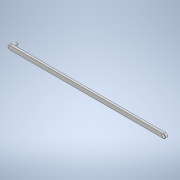
# Autodesk Inventor part: eslabon_1
Saved by Autodesk Inventor 2021 (Build 250183000, 183)
## iProperties
Created: 2021-07-12
Part Number: eslabon_1
Material: Genérico
Document SubType Name: Modeling
Designer: Leonardo Fabio Mercado Benítez
Density: 1 g/cm^3
Appearance: Valor por defecto
Author: Leonardo Fabio Mercado Benítez
Autodesk Inventor part; units mm, degrees
ref_plane "YZ Plane" through (0, 0, 0) normal (1, 0, 0) x (0, 1, 0)
ref_plane "XZ Plane" through (0, 0, 0) normal (0, 1, 0) x (-1, 0, 0)
ref_plane "XY Plane" through (0, 0, 0) normal (0, 0, 1) x (1, 0, 0)
sketch "Boceto1" plane through (0, 0, 0) normal (0, 0, 1) x (1, 0, 0)
  arc A0 (0, 3.175) -> (0, -3.175) centre (0, 0) ccw
  arc A1 (240, -3.175) -> (240, 3.175) centre (240, 0) ccw
  line L0 (0, 3.175) -> (240, 3.175)
  line L1 (240, -3.175) -> (0, -3.175)
  dimension "d0" = 6.35
  dimension "d3" = 6.35
  constraints: 4 end point, 4 point on circle, 3 tangent, 2 centre point, 1 coincident
  measures "d0" diameter of A0
  measures "d3" diameter of A1
extrude "Extrusión1" add sketch "Boceto1" along normal blind 3.175
sketch "Boceto2" plane through (0, 0, 0) normal (0, 0, -1) x (-1, 0, 0)
  circle A0 centre (0, 0) radius 2.175
  constraints: 1 centre point, 1 coincident
extrude "Extrusión2" add sketch "Boceto2" along normal blind 7
sketch "Boceto3" plane through (0, 0, 3.175) normal (0, 0, 1) x (1, 0, 0)
  arc A0 (240, -3.175) -> (240, 3.175) centre (240, 0) ccw projected
  circle A1 centre (240, 0) radius 3.175
  circle A2 centre (240, 0) radius 2.675
  point P0 (0, 0)
  dimension "d10" = 6.35
  dimension "d11" = 0.5
  constraints: 2 centre point, 1 coincident
  measures "d10" diameter of A1
  measures "d11" radial gap between concentric circles of A1 A2
extrude "Extrusión3" cut sketch "Boceto3" against normal blind 5 contours A2
